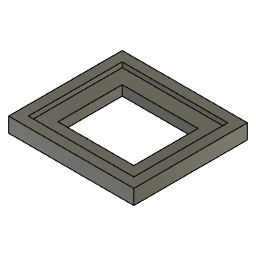
Sensor_Housing (Autodesk Fusion 360 archive; units mm, degrees)
design "Base_Plate_Lens v1"
Autodesk Fusion 360 part; units mm, degrees
sketch "BasePlate" plane through (0, 0, 0) normal (0, 0, 1) x (1, 0, 0)
  line L0 (21.35, 9.5) -> (0, 9.5)
  line L1 (21.35, 9.5) -> (21.35, -9.5)
  line L2 (0, -9.5) -> (0, 9.5)
  line L3 (0, -9.5) -> (21.35, -9.5)
  line L4 (-2, 11.5) -> (23.35, 11.5)
  line L5 (23.35, 11.5) -> (23.35, -11.5)
  line L6 (23.35, -11.5) -> (-2, -11.5)
  line L7 (-2, -11.5) -> (-2, 11.5)
  line L8 (3, 6.5) -> (18.35, 6.5)
  line L9 (18.35, 6.5) -> (18.35, -6.5)
  line L10 (18.35, -6.5) -> (3, -6.5)
  line L11 (3, -6.5) -> (3, 6.5)
  dimension "d4" = 21.35
  dimension "d13" = 19
  constraint horizontal L0
  constraint vertical L1
  constraint vertical L2
  constraint horizontal L4
  constraint vertical L5
  constraint horizontal L6
  constraint vertical L7
  constraint horizontal L8
  constraint vertical L9
  constraint horizontal L10
  constraint vertical L11
  measures "d4" distance of L1.end L2.start
  measures "d13" distance of L1.end L0.start
extrude "Extrude1" add sketch "BasePlate" along normal blind 2 contours L0 L1 L2 L3
extrude "Extrude2" add sketch "BasePlate" along normal blind 3 contours L4 L5 L6 L7
